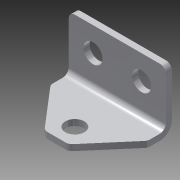
# Autodesk Inventor part: Flange for Torsion Spring
Saved by Autodesk Inventor 2014 (Build 180170000, 170)
## iProperties
Created: 2014-01-05
Part Number: Flange for Torsion Spring
Material: Aluminum
Document SubType Name: Sheet Metal
Designer: Michael
Density: 2.71 g/cm^3
Sheet Metal Rule: Default
Appearance: Satin
Mass: 2.64555 g
Surface Area: 14.6091 cm^2
Volume: 0.976219 cm^3
Author: Michael
Autodesk Inventor part; units mm, degrees
ref_plane "YZ Plane" through (0, 0, 0) normal (1, 0, 0) x (0, 1, 0)
ref_plane "XZ Plane" through (0, 0, 0) normal (0, 1, 0) x (-1, 0, 0)
ref_plane "XY Plane" through (0, 0, 0) normal (0, 0, 1) x (1, 0, 0)
sketch "Sketch1" plane through (0, 0, 0) normal (0, 0, 1) x (1, 0, 0)
  line L0 (0, 0) -> (25.4, 0)
  line L1 (25.4, 0) -> (25.4, 12.7)
  line L2 (25.4, 12.7) -> (0, 12.7)
  line L3 (0, 12.7) -> (0, 0)
  circle A0 centre (6.35, 6.35) radius 2.4892
  circle A1 centre (19.05, 6.35) radius 2.4892
  line L4 (12.7, 12.7) -> (12.7, 0) construction
  dimension "d0" = 25.4
  dimension "d1" = 12.7
  dimension "d2" = 4.9784
  dimension "d3" = 4.9784
  dimension "d4" = 6.35
  dimension "d5" = 6.35
  dimension "d6" = 6.35
  dimension "d7" = 6.35
  measures "d0" distance of L2.end L1.end
  measures "d1" distance of L1.end L0.end
  measures "d2" diameter of A0
  measures "d3" diameter of A1
  measures "d4" distance from line of L0 A0.centre
  measures "d5" distance from line of L0 A1.centre
  measures "d6" distance from line of L4 A0.centre
  measures "d7" distance from line of A1.centre L4
extrude "Plate1" add sketch "Sketch1" along normal blind 1.5875
sketch "Sketch2" plane through (25.4, -1.5875, 3.175) normal (0, -1, 0) x (1, 0, 0)
  line L0 (-25.4, 0) -> (0, 0)
  line L1 (0, 0) -> (0, 14.2875)
  line L2 (0, 14.2875) -> (-25.4, 14.2875)
  line L3 (-25.4, 14.2875) -> (-25.4, 0)
  constraints: 6 end point, 1 horizontal, 1 perpendicular, 1 vertical
edge flange "Flange1" height 17.4625 angle 90 thickness 1.5875 bend radius 1.5875 thickness toward (0, -1, 0) relief straight relief width 1.5875 relief depth 0.7937 edges at (12.7, 0, 1.5875) wall of the first edge with corners at (0, -1.5875, 3.175) (25.4, -1.5875, 3.175) (25.4, -1.5875, 17.4625) (0, -1.5875, 17.4625)
bend "Bend1"
corner "Corner1"
sketch "Sketch3" plane through (0, -1.5875, 17.4625) normal (0, 1, 0) x (1, 0, 0)
  line L0 (25.4, 14.2875) -> (0, 14.2875) projected
  line L1 (0, 0) -> (0, 14.2875) projected
  line L2 (0, 0) -> (25.4, 0) projected
  line L3 (25.4, 0) -> (25.4, 14.2875) projected
  line L4 (0, 11.1125) -> (9.525, 0)
  line L5 (12.7, 0) -> (12.7, 14.2875) construction
  line L6 (25.4, 11.1125) -> (15.875, 0)
  circle A0 centre (12.7, 4.7625) radius 2.4892
  line L7 (9.525, 0) -> (15.875, 0)
  line L8 (25.4, 11.1125) -> (25.4, 14.2875)
  point P0 (0, 17.4625)
  dimension "d19" = 3.175
  dimension "d20" = 3.175
  dimension "d21" = 4.9784
  dimension "d22" = 4.7625
  constraints: 10 end point, 3 point on line, 2 collinear, 2 midpoint, 2 symmetric about line, 1 centre point
  measures "d19" distance from line of L0 L4.start
  measures "d20" distance from line of L5 L4.end
  measures "d21" diameter of A0
  measures "d22" distance from line of L2 A0.centre
extrude "Extrusion1" cut sketch "Sketch3" against normal blind 25.4 contours L3 L2 L6 | L4 L2 L1 | A0
fillet "Fillet1" radius 1.5875 6 edges at (9.525, -2.3812, 17.4625) (0, -2.3813, 6.35) (25.4, -2.3813, 6.35) (15.875, -2.3812, 17.4625) (25.4, 12.7, 0.7937) (0, 12.7, 0.7937)
equation "\"d5\" = d4"
equation "\"d7\" = d6"
equation "\"d9\" = BendReliefWidth"
equation "\"d10\" = BendReliefDepth"
equation "\"d11\" = MinimumRemnant"
equation "\"d12\" = BendRadius"
equation "\"d15\" = BendRadius"
equation "\"d16\" = CornerReliefSize"
equation "\"d17\" = GapSize"
equation "\"d18\" = JacobiRadiusSize"
equation "\"BendRadius\" = Thickness"
equation "\"BendReliefWidth\" = Thickness"
equation "\"BendReliefDepth\" = 0.5 * Thickness"
equation "\"CornerReliefSize\" = 4 * Thickness"
equation "\"MinimumRemnant\" = 2 * Thickness"
equation "\"TransitionRadius\" = BendRadius"
equation "\"JacobiRadiusSize\" = BendRadius"
equation "\"GapSize\" = Thickness"
equation "\"d8\" = BendRadius"
equation "\"Thickness\" = 1.5875"
body "Solid1"
